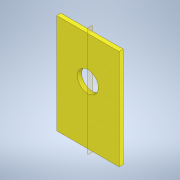
# Autodesk Inventor part: plateForHangingMechanism
Saved by Autodesk Inventor 2020.2 (Build 242310000, 310)
## iProperties
Created: 2020-01-06
Part Number: plateForHangingMechanism
Material: Aluminum 6061
Document SubType Name: Modeling
Designer: steele
Density: 2.7 g/cm^3
Appearance: Canary
Author: steele
Autodesk Inventor part; units mm, degrees
ref_plane "XZ Plane" through (0, 0, 0) normal (0, 1, 0) x (-1, 0, 0)
ref_plane "XY Plane" through (0, 0, 0) normal (0, 0, 1) x (1, 0, 0)
sketch "Sketch1" plane through (0, 0, 0) normal (0, 0, 1) x (1, 0, 0)
  line L0 (-47.625, -76.2) -> (47.625, -76.2)
  line L1 (47.625, -76.2) -> (47.625, 76.2)
  line L2 (47.625, 76.2) -> (-47.625, 76.2)
  line L3 (-47.625, 76.2) -> (-47.625, -76.2)
  line L4 (-47.625, -76.2) -> (47.625, 76.2) construction
  line L5 (47.625, -76.2) -> (-47.625, 76.2) construction
  point P0 (0, 0)
  dimension "d0" = 95.25
  dimension "d1" = 152.4
  constraints: 12 end point, 2 midpoint, 2 parallel, 1 horizontal, 1 perpendicular
  measures "d0" distance of L0.start L0.end
  measures "d1" distance of L1.end L0.end
extrude "Extrusion1" add sketch "Sketch1" against normal blind 6.35
sketch "Sketch2" plane through (0, 0, 0) normal (0, 0, 1) x (1, 0, 0)
  circle A0 centre (0, 12.7) radius 15.875
  line L0 (47.625, 76.2) -> (-47.625, 76.2) projected
  point P0 (0, 0)
  dimension "bearingDiameter" = 31.75
  dimension "d5" = 63.5
  constraints: 1 centre point
  measures "bearingDiameter" diameter of A0
  measures "d5" distance from line of A0.centre L0
extrude "Extrusion2" cut sketch "Sketch2" against normal through all
body "Solid1"
